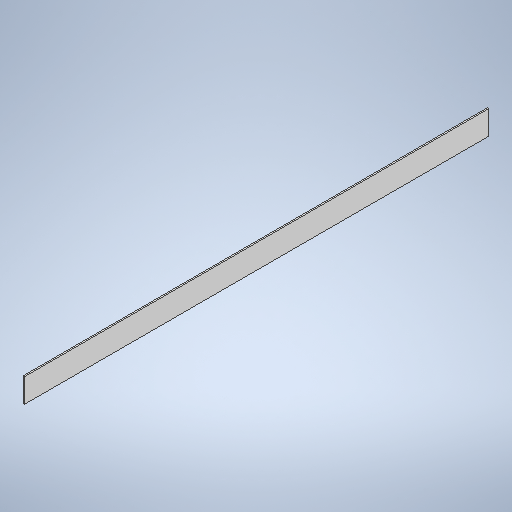
# Autodesk Inventor part: MSC 0692 stringer cone
Saved by Autodesk Inventor 2025 (Build 290162010, 162A)
## iProperties
Created: 2024-06-26
Part Number: MSC 0692 stringer cone
Material: Stainless Steel
Document SubType Name: Sheet Metal
Designer: pokla
Density: 8 g/cm^3
Sheet Metal Rule: AISI304 3mm Die 32
Appearance: Default
Author: pokla
Autodesk Inventor part; units mm, degrees
ref_plane "YZ Plane" through (0, 0, 0) normal (1, 0, 0) x (0, 1, 0)
ref_plane "XZ Plane" through (0, 0, 0) normal (0, 1, 0) x (-1, 0, 0)
ref_plane "XY Plane" through (0, 0, 0) normal (0, 0, 1) x (1, 0, 0)
sketch "Sketch1" plane through (0, 0, 0) normal (0, 0, 1) x (1, 0, 0)
  line L0 (-768, 1124.508) -> (768, 1124.508) construction
  line L1 (-98, 0) -> (98, 0) construction
  line L2 (98, 0) -> (768, 1124.508) construction
  line L3 (-98, 0) -> (-768, 1124.508) construction
  line L4 (-190, 752.254) -> (190, 752.254) construction
  line L5 (190, 752.254) -> (190, 372.254) construction
  line L6 (190, 372.254) -> (-190, 372.254) construction
  line L7 (-190, 372.254) -> (-190, 752.254)
  line L8 (0, 1124.508) -> (0, 0) construction
  line L9 (-190, 752.254) -> (-190, 1124.508)
  line L10 (190, 752.254) -> (190, 1124.508) construction
  line L11 (-190, 372.254) -> (-190, 154.41)
  line L12 (190, 372.254) -> (190, 154.41) construction
  line L13 (-190, 752.254) -> (-546.2051, 752.254) construction
  line L14 (-190, 372.254) -> (-319.7949, 372.254) construction
  line L15 (190, 372.254) -> (319.7949, 372.254) construction
  line L16 (190, 752.254) -> (546.2051, 752.254) construction
  line L17 (-585.0411, 817.4352) -> (-581.9487, 812.2451) construction
  point P0 (0, 752.254)
  point P1 (-190, 562.254)
  point P2 (0, 562.254)
  dimension "d0" = 1536
  dimension "d1" = 196
  dimension "d2" = 1308.976
  dimension "d3" = 380
  dimension "d4" = 380
  measures "d0" distance of L3.end L2.end
  measures "d1" distance of L3.start L2.start
  measures "d2" distance of L2.start L2.end
  measures "d3" distance of L5.end L7.start
  measures "d4" distance of L4.end L5.end
contour flange "Contour Flange1" sketch "Sketch1" thickness 3 bend radius 5 width 50 along (0, 0, 1) mid plane no both sides yes wall seen from (-190, 263.332, 0) lies toward (1, 0, 0) curves L11 L7 L9
bend "Bend1"
corner "Corner1"
equation "\"d7\" = Thickness"
equation "\"d8\" = BendReliefWidth"
equation "\"d9\" = BendReliefDepth"
equation "\"d10\" = MinimumRemnant"
equation "\"d11\" = TransitionRadius"
equation "\"d13\" = BendRadius"
equation "\"d15\" = CornerReliefSize"
equation "\"d16\" = GapSize"
equation "\"d17\" = JacobiRadiusSize"
equation "\"BendReliefWidth\" = Thickness"
equation "\"BendReliefDepth\" = 0.5 * Thickness"
equation "\"CornerReliefSize\" = 4 * Thickness"
equation "\"MinimumRemnant\" = 2 * Thickness"
equation "\"TransitionRadius\" = BendRadius"
equation "\"JacobiRadiusSize\" = BendRadius"
equation "\"GapSize\" = Thickness"
equation "\"Thickness\" = 3"
equation "\"BendRadius\" = 5"
body "Solid1"
